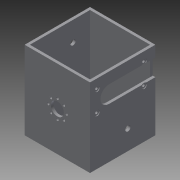
# Autodesk Inventor part: Arm_Bracket_2
Saved by Autodesk Inventor 2013 (Build 170138000, 138)
## iProperties
Created: 2014-04-16
Part Number: Arm_Bracket_2
Material: 一般
Document SubType Name: Modeling
Designer: andou
Density: 1 g/cm^3
Author: andou
Autodesk Inventor part; units mm, degrees
ref_plane "YZ Plane" through (0, 0, 0) normal (1, 0, 0) x (0, 1, 0)
ref_plane "XZ Plane" through (0, 0, 0) normal (0, 1, 0) x (-1, 0, 0)
ref_plane "XY Plane" through (0, 0, 0) normal (0, 0, 1) x (1, 0, 0)
sketch "スケッチ1" plane through (0, 0, 0) normal (0, 0, 1) x (1, 0, 0)
  line L0 (-25, 25) -> (25, 25)
  line L1 (25, 25) -> (25, -25)
  line L2 (25, -25) -> (-25, -25)
  line L3 (-25, -25) -> (-25, 25)
  line L4 (-23, 23) -> (23, 23)
  line L5 (23, 23) -> (23, -23)
  line L6 (23, -23) -> (-23, -23)
  line L7 (-23, -23) -> (-23, 23)
  point P0 (0, 0)
  dimension "d0" = 23
  dimension "d1" = 25
  dimension "d2" = 50
  dimension "d3" = 46
  dimension "d4" = 46
  dimension "d5" = 50
  dimension "d6" = 23
  dimension "d7" = 25
  constraints: 16 end point, 4 parallel, 2 horizontal, 2 perpendicular
  measures "d0" distance from line of point (0, 0) L7
  measures "d1" distance from line of L1 point (0, 0)
  measures "d2" distance of L0.start L0.end
  measures "d3" distance of L4.start L4.end
  measures "d4" distance between parallel lines of L6 L4
  measures "d5" distance between parallel lines of L2 L0
  measures "d6" distance from line of point (0, 0) L6
  measures "d7" distance from line of L0 point (0, 0)
extrude "押し出し1" add sketch "スケッチ1" against normal blind 60
sketch "スケッチ2" plane through (25, -25, 0) normal (1, 0, 0) x (0, 0, -1)
  line L0 (0, 50) -> (0, 0) projected
  line L1 (0, 0) -> (60, 0) projected
  circle A0 centre (15, 35) radius 2
  circle A1 centre (45, 29) radius 2
  point P0 (0, 25)
  dimension "d10" = 4
  dimension "d12" = 30
  dimension "d13" = 15
  dimension "d14" = 6
  dimension "d15" = 29
  constraints: 2 centre point, 1 equal radius
  measures "d10" diameter of A0
  measures "d12" horizontal distance of A1.centre A0.centre
  measures "d13" distance from line of L0 A0.centre
  measures "d14" vertical distance of A0.centre A1.centre
  measures "d15" distance from line of L1 A1.centre
hole "穴1" at (25, 10, -15) at (25, 4, -45) direction (-1, 0, 0) diameter 4 end through all
sketch "スケッチ3" plane through (25, -25, 0) normal (1, 0, 0) x (0, 0, -1)
  circle A0 centre (15, 35) radius 2 projected
  line L0 (0, 50) -> (60, 50) projected
  line L1 (8.5, 50) -> (21.5, 50)
  line L2 (21.5, 50) -> (21.5, 14.5)
  line L3 (8.5, 14.5) -> (8.5, 50)
  arc A1 (8.5, 14.5) -> (21.5, 14.5) centre (15, 14.5) ccw
  circle A2 centre (45, 29) radius 2 projected
  point P0 (0, 25)
  dimension "d23" = 35.5
  dimension "d26" = 13
  dimension "d27" = 6.5
  dimension "d28" = 6.5
  dimension "d74" = 30
  constraints: 6 end point, 2 point on circle, 1 centre point, 1 horizontal, 1 parallel, 1 perpendicular, 1 point on line
  measures "d23" distance from line of L1 A1.centre
  measures "d26" distance between parallel lines of L3 L2
  measures "d27" distance from line of L3 A0.centre
  measures "d28" radius of A1
  measures "d74" horizontal distance of A2.centre A1.centre
extrude "押し出し2" cut sketch "スケッチ3" against normal blind 2 contours L0 L2 A1 L3
sketch "スケッチ4" plane through (25, -25, 0) normal (1, 0, 0) x (0, 0, -1)
  line L0 (0, 50) -> (8.5, 50) projected
  line L1 (21.5, 50) -> (60, 50) projected
  circle A0 centre (7, 41.5) radius 1
  circle A1 centre (7, 5.5) radius 1
  circle A2 centre (23, 41.5) radius 1
  circle A3 centre (23, 5.5) radius 1
  arc A4 (8.5, 14.5) -> (21.5, 14.5) centre (15, 14.5) ccw projected
  point P0 (0, 25)
  dimension "d32" = 8.5
  dimension "d33" = 8.5
  dimension "d34" = 36
  dimension "d35" = 36
  dimension "d36" = 16
  dimension "d37" = 16
  dimension "d40" = 2
  dimension "d72" = 8
  dimension "d73" = 8
  constraints: 4 centre point, 3 equal radius
  measures "d32" distance from line of L0 A0.centre
  measures "d33" distance from line of L1 A2.centre
  measures "d34" distance of A2.centre A3.centre
  measures "d35" distance of A0.centre A1.centre
  measures "d36" distance of A3.centre A1.centre
  measures "d37" distance of A2.centre A0.centre
  measures "d40" diameter of A3
  measures "d72" horizontal distance of A4.centre A0.centre
  measures "d73" horizontal distance of A4.centre A1.centre
hole "穴2" at (25, 16.5, -7) at (25, 16.5, -23) at (25, -19.5, -7) at (25, -19.5, -23) direction (-1, 0, 0) diameter 2 depth 2 tip angle 118 counterbore diameter 4 counterbore depth 0.5
sketch "スケッチ5" plane through (-25, -25, 0) normal (0, -1, 0) x (1, 0, 0)
  line L0 (50, 0) -> (0, 0) projected
  line L1 (0, 0) -> (0, -60) projected
  circle A0 centre (25, -30) radius 5
  point P0 (25, 0)
  dimension "d48" = 25
  dimension "d49" = 30
  dimension "d50" = 10
  constraints: 1 centre point
  measures "d48" distance from line of L1 A0.centre
  measures "d49" distance from line of L0 A0.centre
  measures "d50" diameter of A0
hole "穴3" at (0, -25, -30) direction (0, 1, 0) diameter 10 depth 2 tip angle 118
sketch "スケッチ6" plane through (-25, -25, 0) normal (0, -1, 0) x (1, 0, 0)
  circle A0 centre (25, -30) radius 5 projected
  line L0 (0, 0) -> (0, -60) projected
  circle A1 centre (25, -23) radius 1
  point P0 (25, 0)
  dimension "d58" = 2
  dimension "d60" = 7
  dimension "d61" = 25
  constraints: 1 centre point
  measures "d58" diameter of A1
  measures "d60" distance of A1.centre A0.centre
  measures "d61" distance from line of L0 A1.centre
hole "穴4" at (0, -25, -23) direction (0, 1, 0) diameter 2 depth 2 tip angle 118
pattern_circular "円形状パターン1" count 8 over 360 about axis through (0, -24, -30) along (0, -1, 0) of "穴4"
